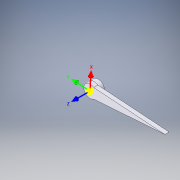
# Autodesk Inventor part: pointer_small
Saved by Autodesk Inventor 2019 (Build 230136000, 136)
## iProperties
Created: 2018-04-29
Part Number: pointer_small
Material: ABS Plastic
Document SubType Name: Modeling
Designer: Fierl
Density: 1.06 g/cm^3
Appearance: Smooth - White
Mass: 0.0308248 g
Surface Area: 0.963841 cm^2
Volume: 0.02908 cm^3
Author: Fierl
Autodesk Inventor part; units mm, degrees
ref_plane "YZ Plane" through (0, 0, 0) normal (1, 0, 0) x (0, 1, 0)
ref_plane "XZ Plane" through (0, 0, 0) normal (0, 1, 0) x (-1, 0, 0)
ref_plane "XY Plane" through (0, 0, 0) normal (0, 0, 1) x (1, 0, 0)
sketch "Sketch1" plane through (0, 0, 0) normal (0, 0, 1) x (1, 0, 0)
  circle A0 centre (0, 0) radius 0.5
  circle A1 centre (0.0161, 0) radius 1.5
  line L0 (-5.3807, 0) -> (21.8968, 0) projected
  line L1 (0.0161, 0) -> (15.0161, 0)
  line L2 (15.0161, 0) -> (18, 0)
  line L3 (18, 0) -> (0.9161, 1.2)
  line L4 (18, 0) -> (0.9161, -1.2)
  dimension "d0" = 1
  dimension "d1" = 3
  dimension "d3" = 2.4
  dimension "d13" = 18
  constraints: 8 end point, 2 centre point, 2 point on circle, 2 point on line, 1 coincident, 1 symmetric about line
  measures "d0" diameter of A0
  measures "d1" diameter of A1
  measures "d3" distance of L4.end L3.end
  measures "d13" distance of point (0, 0) L2.end
extrude "Extrusion1" add sketch "Sketch1" along normal blind 1 contours L0 A1 A0 | A0 L0 A1 | L0 L4 A1 | A1 L3 L0
sketch "Sketch2" plane through (0, 0, 0) normal (0, 0, -1) x (-1, 0, 0)
  circle A0 centre (0, 0) radius 0.5
  circle A1 centre (0.0161, 0) radius 1.5
  line L0 (-5.7839, 0) -> (24.3161, 0)
  line L1 (0.0161, 0) -> (20.0161, 0)
  line L2 (20.0161, 0) -> (20.0155, 0)
  line L3 (20.0155, 0) -> (0.8452, 1.25)
  line L4 (20.0155, 0) -> (0.8452, -1.25)
  dimension "d6" = 1
  dimension "d7" = 3
  dimension "d8" = 20
  dimension "d9" = 2.5
  constraints: 10 end point, 2 centre point, 2 point on circle, 2 point on line, 1 coincident, 1 symmetric about line
  measures "d6" diameter of A0
  measures "d7" diameter of A1
  measures "d8" distance of L1.start L1.end
  measures "d9" distance of L4.end L3.end
extrude "Extrusion2" add sketch "Sketch2" along normal blind 1 contours L0 A1 A0 | A0 L0 A1
equation "\"d0\" = pointer_axis"
equation "\"d1\" = pointer_axis_outside"
equation "\"d3\" = 0.8 * pointer_axis_outside"
equation "\"d13\" = pointer_length"
equation "\"circle_dimension\" = 56"
equation "\"circle_dimension_inner\" = 47"
equation "\"hole_from_center\" = 63.5"
equation "\"hole_distance\" = 22.45064"
equation "\"ring_depth\" = 6"
equation "\"ring_thickness\" = 9"
equation "\"ring_top_thickness\" = 2"
equation "\"ring_outer_bevel_height\" = 3"
equation "\"ring_outer_bevel_depth\" = 0.5"
equation "\"ring_inner_bevel_depth\" = 3.5"
equation "\"screw_distance_center\" = 15"
equation "\"screw_distance_outside\" = 3.5"
equation "\"front_plate_thickness\" = 2"
equation "\"glass_thickness\" = 2"
equation "\"encoders\" = 0"
equation "\"encoder_axis\" = 8"
equation "\"encoder_emboss\" = 0"
equation "\"encoder_width\" = 27"
equation "\"encoder_rad\" = 49"
equation "\"encoder_extrude_hight\" = 3"
equation "\"pointer_axis\" = 1"
equation "\"pointer_axis_outside\" = 3"
equation "\"pointer_length\" = 18"
body "Solid1"
